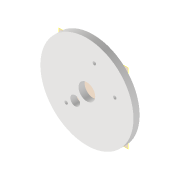
# Autodesk Inventor part: Anglerfish_3inch_tube_adapterplate_focus
Saved by Autodesk Inventor 2022 (Build 260153000, 153)
## iProperties
Created: 2022-04-12
Part Number: Anglerfish_3inch_tube_adapterplate_focus
Material: Generic
Document SubType Name: Modeling
Designer: Prakash Lab
Density: 1 g/cm^3
Appearance: Default
Author: Prakash Lab
Autodesk Inventor part; units mm, degrees
ref_plane "YZ Plane" through (0, 0, 0) normal (1, 0, 0) x (0, 1, 0)
ref_plane "XZ Plane" through (0, 0, 0) normal (0, 1, 0) x (-1, 0, 0)
ref_plane "XY Plane" through (0, 0, 0) normal (0, 0, 1) x (1, 0, 0)
ref_plane "Work Plane1" through (-4.987218, -5.774768, 0) normal (0, 0, 1) x (0.9999987, 0.0016281, 0)
sketch "Sketch1" plane through (-4.987218, -5.774768, 0) normal (0, 0, 1) x (0.9999987, 0.0016281, 0)
  circle A0 centre (0.000199, -0.002158) radius 38.1
  circle A1 centre (0.000199, -0.002158) radius 37.8
  circle A2 centre (-0.048773, -0.058769) radius 6.775396
  circle A3 centre (6.079487, 22.963606) radius 1.4
  circle A4 centre (-16.87798, -16.104757) radius 1.4
  circle A5 centre (22.663033, 7.130604) radius 1.4
  point P0 (4.996614, 5.76664)
  dimension "d0" = 0.3
  constraints: 1 centre point
  measures "d0" radial gap between concentric circles of A0 A1
sketch "Sketch1 outline for Extrusion1" plane through (-4.987218, -5.774768, 0) normal (0, 0, 1) x (0.9999987, 0.0016281, 0)
  circle A0 centre (0.000199, -0.002158) radius 37.8
  circle A1 centre (-16.87798, -16.104757) radius 1.4
  circle A2 centre (-0.048773, -0.058769) radius 6.775396
  circle A3 centre (22.663033, 7.130604) radius 1.4
  circle A4 centre (6.079487, 22.963606) radius 1.4
extrude "Extrusion1" add sketch "Sketch1 outline for Extrusion1" along normal blind 5
sketch "Sketch4" plane through (-4.987218, -5.774768, 5) normal (0, 0, 1) x (0.9999987, 0.0016281, 0)
  circle A0 centre (19.372358, 5.196915) radius 1.4
  circle A1 centre (-9.548696, -11.058773) radius 1.352011
  circle A2 centre (-9.548696, -11.058773) radius 3.95399
  point P0 (4.996614, 5.76664)
  constraints: 1 centre point, 1 coincident
extrude "Extrusion4" cut sketch "Sketch4" against normal blind 25.4 contours A1 | A2
shell "Shell1" thickness 2.54 removed faces 1 at (15.854163, -10.364044, 0)
body "Solid1"
